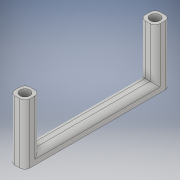
# Autodesk Inventor part: Battery Holder
Saved by Autodesk Inventor 2019 (Build 230136000, 136)
## iProperties
Created: 2018-12-28
Part Number: Battery Holder
Material: Generic
Document SubType Name: Modeling
Designer: ashle
Density: 1 g/cm^3
Appearance: Default
Author: ashle
Autodesk Inventor part; units mm, degrees
ref_plane "YZ Plane" through (0, 0, 0) normal (1, 0, 0) x (0, 1, 0)
ref_plane "XZ Plane" through (0, 0, 0) normal (0, 1, 0) x (-1, 0, 0)
ref_plane "XY Plane" through (0, 0, 0) normal (0, 0, 1) x (1, 0, 0)
sketch "Sketch1" plane through (0, 0, 0) normal (0, 1, 0) x (-1, 0, 0)
  line L0 (-3, -29) -> (3, -29)
  line L1 (3, -29) -> (3, 29)
  line L2 (3, 29) -> (-3, 29)
  line L3 (-3, 29) -> (-3, -29)
  line L4 (-3, -29) -> (3, 29) construction
  line L5 (3, -29) -> (-3, 29) construction
  point P0 (0, 0)
  dimension "d0" = 58
  dimension "d1" = 6
  constraints: 12 end point, 2 midpoint, 2 parallel, 1 horizontal, 1 perpendicular
  measures "d0" distance of L0.end L1.end
  measures "d1" distance of L1.end L2.end
extrude "Main Body Extrusion" add sketch "Sketch1" along normal blind 4
sketch "Sketch2" plane through (0, 4, 0) normal (0, 1, 0) x (1, 0, 0)
  line L0 (-3, 29) -> (-3, -29) projected
  line L1 (3, -29) -> (3, 29) projected
  line L2 (-3, -29) -> (3, -29)
  line L3 (3, -29) -> (3, -23)
  line L4 (3, -23) -> (-3, -23)
  line L5 (-3, -23) -> (-3, -29)
  line L6 (3, 29) -> (-3, 29) projected
  line L7 (-3, 29) -> (3, 29)
  line L8 (3, 29) -> (3, 23)
  line L9 (3, 23) -> (-3, 23)
  line L10 (-3, 23) -> (-3, 29)
  point P0 (0, 0)
  dimension "d4" = 6
  dimension "d5" = 6
  dimension "d6" = 6
  dimension "d7" = 6
  dimension "d8" = 6
  constraints: 16 end point, 4 parallel, 2 horizontal, 2 perpendicular
  measures "d4" distance between parallel lines of L0 L1
  measures "d5" distance of L4.end L3.end
  measures "d6" distance of L3.end L2.end
  measures "d7" distance of L8.end L9.end
  measures "d8" distance of L7.end L8.end
extrude "Side Beams Extrusion" add sketch "Sketch2" along normal blind 20 contours L6 L1 L9 L0 | L4 L1 L2 L0
sketch "Sketch3" plane through (0, 24, 0) normal (0, 1, 0) x (1, 0, 0)
  line L0 (-3, 23) -> (-3, -23) projected
  line L1 (3, -23) -> (3, 23) projected
  circle A0 centre (0, 26) radius 2
  line L2 (-3, 23) -> (3, 23) projected
  line L3 (3, 29) -> (-3, 29) projected
  circle A1 centre (0, -26) radius 2
  line L4 (-3, -29) -> (3, -29) projected
  line L5 (3, -29) -> (3, -23) projected
  point P0 (0, 0)
  dimension "d11" = 6
  dimension "d12" = 4
  dimension "d13" = 3
  dimension "d14" = 6
  dimension "d15" = 3
  dimension "d16" = 4
  dimension "d17" = 3
  dimension "d18" = 3
  constraints: 2 centre point
  measures "d11" distance between parallel lines of L0 L1
  measures "d12" diameter of A0
  measures "d13" distance from line of L2 A0.centre
  measures "d14" distance between parallel lines of L2 L3
  measures "d15" distance from line of L1 A0.centre
  measures "d16" diameter of A1
  measures "d17" distance from line of L4 A1.centre
  measures "d18" distance from line of L5 A1.centre
extrude "Extrusion3" cut sketch "Sketch3" against normal blind 7
fillet "Fillet1" radius 2 10 edges at (-3, 14, -23) (-3, 12, -29) (-3, 4, 0) (3, 4, 0) (-3, 12, 29) (-3, 14, 23) (3, 12, 29) (3, 14, -23) (3, 12, -29) (3, 14, 23)
equation "\"d5\" = d4"
equation "\"d6\" = d4"
equation "\"d7\" = d4"
equation "\"d8\" = d4"
equation "\"d13\" = 0.5 * d14"
equation "\"d15\" = 0.5 * d11"
equation "\"d17\" = d13"
equation "\"d18\" = d15"
body "Solid1"
